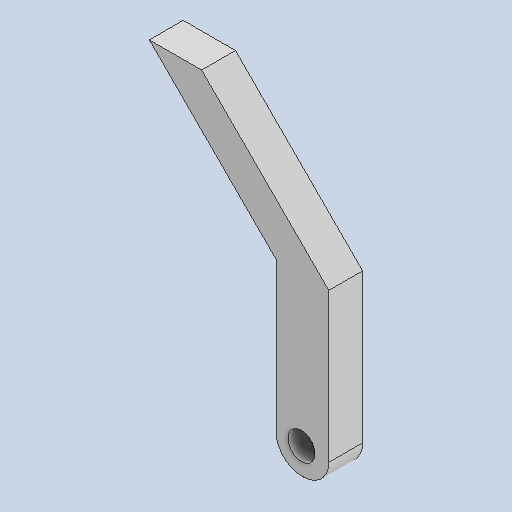
# Autodesk Inventor part: mirror_holder
Saved by Autodesk Inventor 2025.1 (Build 291241020, 241B)
## iProperties
Created: 2024-10-13
Part Number: mirror_holder
Material: Ogólny
Document SubType Name: Modeling
Designer: zychlix
Density: 1 g/cm^3
Appearance: Domyślna
Author: zychlix
Autodesk Inventor part; units mm, degrees
ref_plane "YZ Plane" through (0, 0, 0) normal (1, 0, 0) x (0, 1, 0)
ref_plane "XZ Plane" through (0, 0, 0) normal (0, 1, 0) x (-1, 0, 0)
ref_plane "XY Plane" through (0, 0, 0) normal (0, 0, 1) x (1, 0, 0)
sketch "Szkic1" plane through (0, 0, 0) normal (0, 0, 1) x (1, 0, 0)
  circle A0 centre (3, 5) radius 1.45 projected
  circle A1 centre (3, 5) radius 1.6
  line L0 (6.229, 0) -> (6.229, 8) projected
  line L1 (0, 0) -> (0, 8) projected
  line L2 (3.229, 1.9318) -> (3, 1.9318)
  line L3 (0, 4.9318) -> (0, 22.5946)
  line L4 (6.229, 22.5402) -> (6.229, 4.9318)
  arc A2 (3.229, 1.9318) -> (6.229, 4.9318) centre (3.229, 4.9318) ccw
  arc A3 (0, 4.9318) -> (3, 1.9318) centre (3, 4.9318) ccw
  line L5 (0, 22.5946) -> (-14.9838, 37.5785)
  line L6 (6.229, 22.5402) -> (-8.8092, 37.5785)
  line L7 (-8.8092, 37.5785) -> (-14.9838, 37.5785)
  point P0 (6.229, 1.9318)
  dimension "d0" = 3.2
  dimension "d1" = 3
  dimension "d2" = 135
  constraints: 12 end point, 4 point on circle, 4 point on line, 4 tangent, 3 centre point, 2 horizontal, 2 parallel, 1 coincident, 1 collinear, 1 equal radius, 1 perpendicular
  measures "d0" diameter of A1
  measures "d1" radius of A2
  measures "d2" angle of L3 L5
extrude "Wyciągnięcie proste1" add sketch "Szkic1" along normal blind 4 contours A2 L2 A3 L1 L3 L5 L7 L6 L4 L0
